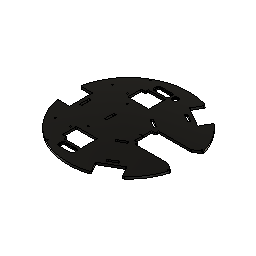
UpperPlate v16 (Autodesk Fusion 360 design; units mm, degrees)
Autodesk Fusion 360 part; units mm, degrees
(part 1 of 2)
sketch "Sketch1" plane through (0, 0, 0) normal (0, 0, 1) x (1, 0, 0)
  line L0 (0, 0) -> (-132.5, 0) construction
  line L1 (0, 0) -> (132.5, 0) construction
  line L2 (0, 0) -> (66.25, 114.7484) construction
  line L3 (0, 0) -> (66.25, -114.7484) construction
  line L4 (-130.1201, -25) -> (-103.7941, -25) construction
  line L5 (-103.7941, -25) -> (-103.7941, 25) construction
  line L6 (-103.7941, 25) -> (-130.1201, 25) construction
  line L7 (-130.1201, 25) -> (-130.1201, -25) construction
  line L8 (-103.7941, 25) -> (-104.8548, 23.9393) construction
  line L9 (-103.7941, -25) -> (-104.8548, -23.9393) construction
  arc A0 (-127.0581, -25) -> (-129.5015, -28.0288) centre (-127.0581, -27.5) ccw
  arc A1 (-129.5015, -28.0288) -> (-127.0581, -25) centre (-127.0581, -27.5) ccw construction
  arc A2 (-103.7941, -25) -> (-103.7941, -22.8787) centre (-104.8548, -23.9393) ccw
  arc A3 (-103.7941, -22.8787) -> (-105.9155, -25) centre (-104.8548, -23.9393) ccw construction
  arc A4 (-105.9155, -25) -> (-103.7941, -25) centre (-104.8548, -23.9393) ccw
  arc A5 (-103.7941, 22.8787) -> (-105.9155, 25) centre (-104.8548, 23.9393) ccw
  arc A6 (-105.9155, 25) -> (-103.7941, 22.8787) centre (-104.8548, 23.9393) ccw construction
  arc A7 (-129.5015, 28.0288) -> (-127.0581, 25) centre (-127.0581, 27.5) ccw
  arc A8 (-127.0581, 25) -> (-129.5015, 28.0288) centre (-127.0581, 27.5) ccw construction
  line L10 (-127.0581, 25) -> (-105.9155, 25)
  line L11 (-103.7941, 22.8787) -> (-103.7941, -22.8787)
  line L12 (-105.9155, -25) -> (-127.0581, -25)
  line L13 (43.4094, 125.1873) -> (86.7107, 100.1873) construction
  line L14 (43.4094, 125.1873) -> (30.2464, 102.3884) construction
  line L15 (30.2464, 102.3884) -> (73.5477, 77.3884) construction
  line L16 (73.5477, 77.3884) -> (86.7107, 100.1873) construction
  arc A9 (41.8784, 122.5355) -> (40.477, 126.166) centre (39.7133, 123.7855) ccw
  arc A10 (40.477, 126.166) -> (41.8784, 122.5355) centre (39.7133, 123.7855) ccw construction
  arc A11 (89.0244, 98.1371) -> (85.1797, 97.5355) centre (87.3447, 96.2855) ccw
  arc A12 (85.1797, 97.5355) -> (89.0244, 98.1371) centre (87.3447, 96.2855) ccw construction
  line L17 (30.2464, 102.3884) -> (31.6953, 102.7766) construction
  arc A13 (31.3071, 104.2255) -> (32.0836, 101.3277) centre (31.6953, 102.7766) ccw
  arc A14 (32.0836, 101.3277) -> (31.3071, 104.2255) centre (31.6953, 102.7766) ccw construction
  line L18 (73.5477, 77.3884) -> (73.1595, 78.8372) construction
  arc A15 (71.7106, 78.449) -> (74.6084, 79.2255) centre (73.1595, 78.8372) ccw
  arc A16 (74.6084, 79.2255) -> (71.7106, 78.449) centre (73.1595, 78.8372) ccw construction
  line L19 (74.6084, 79.2255) -> (85.1797, 97.5355)
  line L20 (71.7106, 78.449) -> (32.0836, 101.3277)
  line L21 (31.3071, 104.2255) -> (41.8784, 122.5355)
  line L22 (43.4094, -125.1873) -> (86.7107, -100.1873) construction
  line L23 (43.4094, -125.1873) -> (30.2464, -102.3884) construction
  line L24 (30.2464, -102.3884) -> (73.5477, -77.3884) construction
  line L25 (73.5477, -77.3884) -> (86.7107, -100.1873) construction
  line L26 (73.5477, -77.3884) -> (73.1595, -78.8372) construction
  line L27 (30.2464, -102.3884) -> (31.6953, -102.7766) construction
  arc A17 (32.0836, -101.3277) -> (31.3071, -104.2255) centre (31.6953, -102.7766) ccw
  arc A18 (31.3071, -104.2255) -> (32.0836, -101.3277) centre (31.6953, -102.7766) ccw construction
  arc A19 (74.6084, -79.2255) -> (71.7106, -78.449) centre (73.1595, -78.8372) ccw
  arc A20 (71.7106, -78.449) -> (74.6084, -79.2255) centre (73.1595, -78.8372) ccw construction
  arc A21 (85.1797, -97.5355) -> (89.0244, -98.1371) centre (87.3447, -96.2855) ccw
  arc A22 (89.0244, -98.1371) -> (85.1797, -97.5355) centre (87.3447, -96.2855) ccw construction
  arc A23 (40.477, -126.166) -> (41.8784, -122.5355) centre (39.7133, -123.7855) ccw
  arc A24 (41.8784, -122.5355) -> (40.477, -126.166) centre (39.7133, -123.7855) ccw construction
  line L28 (85.1797, -97.5355) -> (74.6084, -79.2255)
  line L29 (71.7106, -78.449) -> (32.0836, -101.3277)
  line L30 (31.3071, -104.2255) -> (41.8784, -122.5355)
  arc A25 (40.477, 126.166) -> (-129.5015, 28.0288) centre (0, 0) ccw
  arc A26 (-129.5015, 28.0288) -> (-129.5015, -28.0288) centre (0, 0) ccw construction
  arc A27 (40.477, -126.166) -> (40.477, 126.166) centre (0, 0) ccw construction
  arc A28 (-129.5015, -28.0288) -> (40.477, -126.166) centre (0, 0) ccw
  line L31 (-103.7941, 18.4) -> (-19.3941, 18.4) construction
  line L32 (-19.3941, 18.4) -> (-19.3941, -18.4) construction
  line L33 (-19.3941, -18.4) -> (-103.7941, -18.4) construction
  line L34 (-96.7941, 10) -> (-91.9941, 10) construction
  line L35 (-91.9941, 10) -> (-91.9941, -10) construction
  line L36 (-91.9941, -10) -> (-96.7941, -10) construction
  line L37 (-96.7941, -10) -> (-96.7941, 10) construction
  line L38 (-96.7941, 10) -> (-91.9941, -10) construction
  line L39 (-41.9941, 10) -> (-37.1941, 10) construction
  line L40 (-37.1941, 10) -> (-37.1941, -10) construction
  line L41 (-37.1941, -10) -> (-41.9941, -10) construction
  line L42 (-41.9941, -10) -> (-41.9941, 10) construction
  line L43 (-41.9941, 10) -> (-37.1941, -10) construction
  line L44 (-96.7941, 10) -> (-95.7335, 8.9393) construction
  line L45 (-91.9941, 10) -> (-93.0548, 8.9393) construction
  line L46 (-96.7941, -10) -> (-95.7335, -8.9393) construction
  line L47 (-91.9941, -10) -> (-93.0548, -8.9393) construction
  arc A29 (-94.1155, 10) -> (-91.9941, 7.8787) centre (-93.0548, 8.9393) ccw construction
  arc A30 (-91.9941, 7.8787) -> (-91.9941, 10) centre (-93.0548, 8.9393) ccw
  arc A31 (-91.9941, 10) -> (-94.1155, 10) centre (-93.0548, 8.9393) ccw
  arc A32 (-96.7941, 7.8787) -> (-94.6728, 10) centre (-95.7335, 8.9393) ccw construction
  arc A33 (-94.6728, 10) -> (-96.7941, 10) centre (-95.7335, 8.9393) ccw
  arc A34 (-96.7941, 10) -> (-96.7941, 7.8787) centre (-95.7335, 8.9393) ccw
  arc A35 (-94.6728, -10) -> (-96.7941, -7.8787) centre (-95.7335, -8.9393) ccw construction
  arc A36 (-96.7941, -7.8787) -> (-96.7941, -10) centre (-95.7335, -8.9393) ccw
  arc A37 (-96.7941, -10) -> (-94.6728, -10) centre (-95.7335, -8.9393) ccw
  arc A38 (-91.9941, -7.8787) -> (-94.1155, -10) centre (-93.0548, -8.9393) ccw construction
  arc A39 (-94.1155, -10) -> (-91.9941, -10) centre (-93.0548, -8.9393) ccw
  arc A40 (-91.9941, -10) -> (-91.9941, -7.8787) centre (-93.0548, -8.9393) ccw
  line L48 (-94.6728, 10) -> (-94.1155, 10)
  line L49 (-96.7941, 7.8787) -> (-96.7941, -7.8787)
  line L50 (-91.9941, -7.8787) -> (-91.9941, 7.8787)
  line L51 (-94.6728, -10) -> (-94.1155, -10)
  line L52 (-41.9941, 10) -> (-40.9335, 8.9393) construction
  line L53 (-37.1941, 10) -> (-38.2548, 8.9393) construction
  line L54 (-41.9941, -10) -> (-40.9335, -8.9393) construction
  line L55 (-37.1941, -10) -> (-38.2548, -8.9393) construction
  arc A41 (-37.1941, -7.8787) -> (-39.3155, -10) centre (-38.2548, -8.9393) ccw construction
  arc A42 (-39.3155, -10) -> (-37.1941, -10) centre (-38.2548, -8.9393) ccw
  arc A43 (-37.1941, -10) -> (-37.1941, -7.8787) centre (-38.2548, -8.9393) ccw
  arc A44 (-39.8728, -10) -> (-41.9941, -7.8787) centre (-40.9335, -8.9393) ccw construction
  arc A45 (-41.9941, -10) -> (-39.8728, -10) centre (-40.9335, -8.9393) ccw
  arc A46 (-41.9941, -7.8787) -> (-41.9941, -10) centre (-40.9335, -8.9393) ccw
  arc A47 (-41.9941, 7.8787) -> (-39.8728, 10) centre (-40.9335, 8.9393) ccw construction
  arc A48 (-41.9941, 10) -> (-41.9941, 7.8787) centre (-40.9335, 8.9393) ccw
  arc A49 (-39.8728, 10) -> (-41.9941, 10) centre (-40.9335, 8.9393) ccw
  arc A50 (-39.3155, 10) -> (-37.1941, 7.8787) centre (-38.2548, 8.9393) ccw construction
  arc A51 (-37.1941, 10) -> (-39.3155, 10) centre (-38.2548, 8.9393) ccw
  arc A52 (-37.1941, 7.8787) -> (-37.1941, 10) centre (-38.2548, 8.9393) ccw
  line L56 (-39.8728, -10) -> (-39.3155, -10)
  line L57 (-37.1941, -7.8787) -> (-37.1941, 7.8787)
  line L58 (-41.9941, 7.8787) -> (-41.9941, -7.8787)
  line L59 (-39.8728, 10) -> (-39.3155, 10)
  line L60 (35.9622, 99.0884) -> (-6.2378, 25.9958) construction
  line L61 (-6.2378, 25.9958) -> (25.6319, 7.5958) construction
  line L62 (25.6319, 7.5958) -> (67.8319, 80.6884) construction
  line L63 (39.7368, 88.8262) -> (57.0573, 78.8262) construction
  line L64 (57.0573, 78.8262) -> (54.6573, 74.6693) construction
  line L65 (54.6573, 74.6693) -> (37.3368, 84.6693) construction
  line L66 (37.3368, 84.6693) -> (39.7368, 88.8262) construction
  line L67 (39.7368, 88.8262) -> (54.6573, 74.6693) construction
  line L68 (12.3368, 41.368) -> (29.6573, 31.368) construction
  line L69 (29.6573, 31.368) -> (27.2573, 27.2111) construction
  line L70 (27.2573, 27.2111) -> (9.9368, 37.2111) construction
  line L71 (9.9368, 37.2111) -> (12.3368, 41.368) construction
  line L72 (12.3368, 41.368) -> (27.2573, 27.2111) construction
  line L73 (37.3368, 84.6693) -> (38.7857, 85.0575) construction
  line L74 (39.7368, 88.8262) -> (40.125, 87.3773) construction
  line L75 (54.6573, 74.6693) -> (54.2691, 76.1181) construction
  line L76 (57.0573, 78.8262) -> (55.6084, 78.438) construction
  arc A53 (55.2202, 79.8868) -> (55.9967, 76.9891) centre (55.6084, 78.438) ccw construction
  arc A54 (55.9967, 76.9891) -> (57.0573, 78.8262) centre (55.6084, 78.438) ccw
  arc A55 (57.0573, 78.8262) -> (55.2202, 79.8868) centre (55.6084, 78.438) ccw
  arc A56 (55.718, 76.5064) -> (52.8202, 75.7299) centre (54.2691, 76.1181) ccw construction
  arc A57 (54.6573, 74.6693) -> (55.718, 76.5064) centre (54.2691, 76.1181) ccw
  arc A58 (52.8202, 75.7299) -> (54.6573, 74.6693) centre (54.2691, 76.1181) ccw
  arc A59 (39.1739, 83.6086) -> (38.3975, 86.5064) centre (38.7857, 85.0575) ccw construction
  arc A60 (37.3368, 84.6693) -> (39.1739, 83.6086) centre (38.7857, 85.0575) ccw
  arc A61 (38.3975, 86.5064) -> (37.3368, 84.6693) centre (38.7857, 85.0575) ccw
  arc A62 (38.6762, 86.9891) -> (41.5739, 87.7655) centre (40.125, 87.3773) ccw construction
  arc A63 (41.5739, 87.7655) -> (39.7368, 88.8262) centre (40.125, 87.3773) ccw
  arc A64 (39.7368, 88.8262) -> (38.6762, 86.9891) centre (40.125, 87.3773) ccw
  line L77 (38.3975, 86.5064) -> (38.6762, 86.9891)
  line L78 (41.5739, 87.7655) -> (55.2202, 79.8868)
  line L79 (55.9967, 76.9891) -> (55.718, 76.5064)
  line L80 (52.8202, 75.7299) -> (39.1739, 83.6086)
  line L81 (9.9368, 37.2111) -> (11.3857, 37.5993) construction
  line L82 (12.3368, 41.368) -> (12.725, 39.9191) construction
  line L83 (27.2573, 27.2111) -> (26.8691, 28.66) construction
  line L84 (29.6573, 31.368) -> (28.2084, 30.9798) construction
  arc A65 (11.2762, 39.5309) -> (14.1739, 40.3073) centre (12.725, 39.9191) ccw construction
  arc A66 (14.1739, 40.3073) -> (12.3368, 41.368) centre (12.725, 39.9191) ccw
  arc A67 (12.3368, 41.368) -> (11.2762, 39.5309) centre (12.725, 39.9191) ccw
  arc A68 (11.7739, 36.1504) -> (10.9975, 39.0482) centre (11.3857, 37.5993) ccw construction
  arc A69 (10.9975, 39.0482) -> (9.9368, 37.2111) centre (11.3857, 37.5993) ccw
  arc A70 (9.9368, 37.2111) -> (11.7739, 36.1504) centre (11.3857, 37.5993) ccw
  arc A71 (28.318, 29.0482) -> (25.4202, 28.2717) centre (26.8691, 28.66) ccw construction
  arc A72 (25.4202, 28.2717) -> (27.2573, 27.2111) centre (26.8691, 28.66) ccw
  arc A73 (27.2573, 27.2111) -> (28.318, 29.0482) centre (26.8691, 28.66) ccw
  arc A74 (27.8202, 32.4286) -> (28.5967, 29.5309) centre (28.2084, 30.9798) ccw construction
  arc A75 (28.5967, 29.5309) -> (29.6573, 31.368) centre (28.2084, 30.9798) ccw
  arc A76 (29.6573, 31.368) -> (27.8202, 32.4286) centre (28.2084, 30.9798) ccw
  line L85 (10.9975, 39.0482) -> (11.2762, 39.5309)
  line L86 (11.7739, 36.1504) -> (25.4202, 28.2717)
  line L87 (28.318, 29.0482) -> (28.5967, 29.5309)
  line L88 (27.8202, 32.4286) -> (14.1739, 40.3073)
  line L89 (35.9622, -99.0884) -> (-6.2378, -25.9958) construction
  line L90 (-6.2378, -25.9958) -> (25.6319, -7.5958) construction
  line L91 (25.6319, -7.5958) -> (67.8319, -80.6884) construction
  line L92 (39.7368, -88.8262) -> (57.0573, -78.8262) construction
  line L93 (57.0573, -78.8262) -> (54.6573, -74.6693) construction
  line L94 (54.6573, -74.6693) -> (37.3368, -84.6693) construction
  line L95 (37.3368, -84.6693) -> (39.7368, -88.8262) construction
  line L96 (37.3368, -84.6693) -> (57.0573, -78.8262) construction
  line L97 (12.3368, -41.368) -> (29.6573, -31.368) construction
  line L98 (29.6573, -31.368) -> (27.2573, -27.2111) construction
  line L99 (27.2573, -27.2111) -> (9.9368, -37.2111) construction
  line L100 (9.9368, -37.2111) -> (12.3368, -41.368) construction
  line L101 (9.9368, -37.2111) -> (29.6573, -31.368) construction
  line L102 (9.9368, -37.2111) -> (11.3857, -37.5993) construction
  line L103 (12.3368, -41.368) -> (12.725, -39.9191) construction
  line L104 (27.2573, -27.2111) -> (26.8691, -28.66) construction
  line L105 (29.6573, -31.368) -> (28.2084, -30.9798) construction
  arc A77 (25.4202, -28.2717) -> (28.318, -29.0482) centre (26.8691, -28.66) ccw construction
  arc A78 (28.318, -29.0482) -> (27.2573, -27.2111) centre (26.8691, -28.66) ccw
  arc A79 (27.2573, -27.2111) -> (25.4202, -28.2717) centre (26.8691, -28.66) ccw
  arc A80 (28.5967, -29.5309) -> (27.8202, -32.4286) centre (28.2084, -30.9798) ccw construction
  arc A81 (29.6573, -31.368) -> (28.5967, -29.5309) centre (28.2084, -30.9798) ccw
  arc A82 (27.8202, -32.4286) -> (29.6573, -31.368) centre (28.2084, -30.9798) ccw
  arc A83 (14.1739, -40.3073) -> (11.2762, -39.5309) centre (12.725, -39.9191) ccw construction
  arc A84 (12.3368, -41.368) -> (14.1739, -40.3073) centre (12.725, -39.9191) ccw
  arc A85 (11.2762, -39.5309) -> (12.3368, -41.368) centre (12.725, -39.9191) ccw
  arc A86 (10.9975, -39.0482) -> (11.7739, -36.1504) centre (11.3857, -37.5993) ccw construction
  arc A87 (9.9368, -37.2111) -> (10.9975, -39.0482) centre (11.3857, -37.5993) ccw
  arc A88 (11.7739, -36.1504) -> (9.9368, -37.2111) centre (11.3857, -37.5993) ccw
  line L106 (28.5967, -29.5309) -> (28.318, -29.0482)
  line L107 (25.4202, -28.2717) -> (11.7739, -36.1504)
  line L108 (27.8202, -32.4286) -> (14.1739, -40.3073)
  line L109 (11.2762, -39.5309) -> (10.9975, -39.0482)
  line L110 (37.3368, -84.6693) -> (38.7857, -85.0575) construction
  line L111 (39.7368, -88.8262) -> (40.125, -87.3773) construction
  line L112 (54.6573, -74.6693) -> (54.2691, -76.1181) construction
  line L113 (57.0573, -78.8262) -> (55.6084, -78.438) construction
  arc A89 (38.3975, -86.5064) -> (39.1739, -83.6086) centre (38.7857, -85.0575) ccw construction
  arc A90 (39.1739, -83.6086) -> (37.3368, -84.6693) centre (38.7857, -85.0575) ccw
  arc A91 (37.3368, -84.6693) -> (38.3975, -86.5064) centre (38.7857, -85.0575) ccw
  arc A92 (41.5739, -87.7655) -> (38.6762, -86.9891) centre (40.125, -87.3773) ccw construction
  arc A93 (38.6762, -86.9891) -> (39.7368, -88.8262) centre (40.125, -87.3773) ccw
  arc A94 (39.7368, -88.8262) -> (41.5739, -87.7655) centre (40.125, -87.3773) ccw
  arc A95 (55.9967, -76.9891) -> (55.2202, -79.8868) centre (55.6084, -78.438) ccw construction
  arc A96 (55.2202, -79.8868) -> (57.0573, -78.8262) centre (55.6084, -78.438) ccw
  arc A97 (57.0573, -78.8262) -> (55.9967, -76.9891) centre (55.6084, -78.438) ccw
  arc A98 (52.8202, -75.7299) -> (55.718, -76.5064) centre (54.2691, -76.1181) ccw construction
  arc A99 (55.718, -76.5064) -> (54.6573, -74.6693) centre (54.2691, -76.1181) ccw
  arc A100 (54.6573, -74.6693) -> (52.8202, -75.7299) centre (54.2691, -76.1181) ccw
  line L114 (38.6762, -86.9891) -> (38.3975, -86.5064)
  line L115 (39.1739, -83.6086) -> (52.8202, -75.7299)
  line L116 (55.718, -76.5064) -> (55.9967, -76.9891)
  line L117 (55.2202, -79.8868) -> (41.5739, -87.7655)
  line L118 (32, 18.3) -> (131.2302, 18.3) construction
  line L119 (131.2302, 18.3) -> (131.2302, -18.3) construction
  line L120 (131.2302, -18.3) -> (32, -18.3) construction
  line L121 (32, -18.3) -> (32, 18.3) construction
  line L122 (40, 25.5) -> (130.0231, 25.5) construction
  line L123 (130.0231, 25.5) -> (130.0231, -25.5) construction
  line L124 (130.0231, -25.5) -> (40, -25.5) construction
  line L125 (40, -25.5) -> (40, 25.5) construction
  line L126 (105, 25.5) -> (105, -25.5) construction
  line L127 (105, 22.5) -> (127.6365, 35.5692) construction
  line L128 (105, -22.5) -> (127.6365, -35.5692) construction
  line L129 (32, -18.3) -> (33.0607, -17.2393) construction
  line L130 (40, -25.5) -> (41.0607, -24.4393) construction
  circle A101 centre (33.0607, -17.2393) radius 1.5 construction
  circle A102 centre (41.0607, -24.4393) radius 1.5 construction
  circle A103 centre (37.5, -20.8) radius 2.5 construction
  line L131 (32, 18.3) -> (33.0607, 17.2393) construction
  line L132 (40, 25.5) -> (41.0607, 24.4393) construction
  circle A104 centre (41.0607, 24.4393) radius 1.5 construction
  circle A105 centre (33.0607, 17.2393) radius 1.5 construction
  circle A106 centre (37.5, 20.8) radius 2.5 construction
  circle A107 centre (124.6951, -36.7577) radius 2.5 construction
  circle A108 centre (124.6951, 36.7577) radius 2.5 construction
  circle A109 centre (109.5263, 28) radius 2.5 construction
  circle A110 centre (109.5263, -28) radius 2.5 construction
  line L133 (32, 16.1787) -> (32, -16.1787)
  line L134 (34.1213, -18.3) -> (37.5, -18.3)
  line L135 (40, -20.8) -> (40, -23.3787)
  line L136 (42.1213, -25.5) -> (109.5263, -25.5)
  line L137 (110.7763, -25.8349) -> (125.9451, -34.5927)
  line L138 (34.1213, 18.3) -> (37.5, 18.3)
  line L139 (40, 20.8) -> (40, 23.3787)
  line L140 (42.1213, 25.5) -> (109.5263, 25.5)
  line L141 (110.7763, 25.8349) -> (125.9451, 34.5927)
  arc A111 (34.1213, 18.3) -> (32, 16.1787) centre (33.0607, 17.2393) ccw
  arc A112 (42.1213, 25.5) -> (40, 23.3787) centre (41.0607, 24.4393) ccw
  arc A113 (32, -16.1787) -> (34.1213, -18.3) centre (33.0607, -17.2393) ccw
  arc A114 (40, -23.3787) -> (42.1213, -25.5) centre (41.0607, -24.4393) ccw
  arc A115 (37.5, 18.3) -> (40, 20.8) centre (37.5, 20.8) ccw
  arc A116 (40, -20.8) -> (37.5, -18.3) centre (37.5, -20.8) ccw
  arc A117 (109.5263, 25.5) -> (110.7763, 25.8349) centre (109.5263, 28) ccw
  arc A118 (110.7763, -25.8349) -> (109.5263, -25.5) centre (109.5263, -28) ccw
  line L142 (0, 0) -> (124.6951, -36.7577) construction
  line L143 (124.6951, -36.7577) -> (127.0931, -37.4646) construction
  arc A119 (127.0931, -37.4646) -> (125.9451, -34.5927) centre (124.6951, -36.7577) ccw
  line L144 (0, 0) -> (124.6951, 36.7577) construction
  line L145 (124.6951, 36.7577) -> (127.0931, 37.4646) construction
  arc A120 (125.9451, 34.5927) -> (127.0931, 37.4646) centre (124.6951, 36.7577) ccw
  arc A121 (89.0244, -98.1371) -> (127.0931, -37.4646) centre (0, 0) ccw
  arc A122 (127.0931, 37.4646) -> (89.0244, 98.1371) centre (0, 0) ccw
  line L146 (127.6365, -35.5692) -> (123.5112, -37.2289) construction
  circle A123 centre (123.5112, -37.2289) radius 3.5 construction
  circle A124 centre (123.5112, -37.2289) radius 1.5
  line L147 (86.7107, -100.1873) -> (87.5879, -94.7067) construction
  circle A125 centre (87.5879, -94.7067) radius 3.5 construction
  circle A126 centre (87.5879, -94.7067) radius 1.5 construction
  line L148 (43.4094, -125.1873) -> (38.2245, -123.2067) construction
  circle A127 centre (38.2245, -123.2067) radius 3.5 construction
  circle A128 centre (38.2245, -123.2067) radius 1.5 construction
  line L149 (-130.1201, -25) -> (-125.8124, -28.5) construction
  circle A129 centre (-125.8124, -28.5) radius 3.5 construction
  circle A130 centre (-125.8124, -28.5) radius 1.5 construction
  line L150 (-130.1201, 25) -> (-125.8124, 28.5) construction
  circle A131 centre (-125.8124, 28.5) radius 3.5 construction
  circle A132 centre (-125.8124, 28.5) radius 1.5 construction
  line L151 (43.4094, 125.1873) -> (38.2245, 123.2067) construction
  circle A133 centre (38.2245, 123.2067) radius 3.5 construction
  circle A134 centre (38.2245, 123.2067) radius 1.5 construction
  line L152 (86.7107, 100.1873) -> (87.5879, 94.7067) construction
  circle A135 centre (87.5879, 94.7067) radius 3.5 construction
  circle A136 centre (87.5879, 94.7067) radius 1.5 construction
  line L153 (127.6365, 35.5692) -> (123.5112, 37.2289) construction
  circle A137 centre (123.5112, 37.2289) radius 3.5 construction
  circle A138 centre (123.5112, 37.2289) radius 1.5
  line L154 (-125.8124, -28.5) -> (38.2245, -123.2067) construction
  line L155 (-125.8124, 28.5) -> (38.2245, 123.2067) construction
  line L156 (0, 0) -> (-43.794, -75.8534) construction
  line L157 (-43.794, -75.8534) -> (-64.5, -111.7173) construction
  circle A139 centre (-64.5, -111.7173) radius 3.5 construction
  circle A140 centre (-64.5, -111.7173) radius 1.5
  line L158 (0, 0) -> (-43.794, 75.8534) construction
  line L159 (-43.794, 75.8534) -> (-64.5, 111.7173) construction
  circle A141 centre (-64.5, 111.7173) radius 3.5 construction
  circle A142 centre (-64.5, 111.7173) radius 1.5
  line L160 (32.0836, -101.3277) -> (21.5862, -107.3884) construction
  line L161 (21.5862, -107.3884) -> (33.586, -128.1727) construction
  circle A143 centre (28.2185, -125.8758) radius 3.5 construction
  circle A144 centre (28.2185, -125.8758) radius 1.5
  line L162 (71.7106, -78.449) -> (82.208, -72.3884) construction
  line L163 (82.208, -72.3884) -> (94.2078, -93.1727) construction
  circle A145 centre (94.9024, -87.3758) radius 3.5 construction
  line L164 (-103.7941, -25) -> (-103.7941, -35) construction
  line L165 (-103.7941, -35) -> (-127.7938, -35) construction
  circle A146 centre (-123.1209, -38.5) radius 3.5 construction
  line L166 (-103.7941, 25) -> (-103.7941, 35) construction
  line L167 (-103.7941, 35) -> (-127.7938, 35) construction
  circle A147 centre (-123.1209, 38.5) radius 3.5 construction
  line L168 (30.2464, 102.3884) -> (21.5862, 107.3884) construction
  line L169 (21.5862, 107.3884) -> (33.586, 128.1727) construction
  circle A148 centre (28.2185, 125.8758) radius 3.5 construction
  line L170 (73.5477, 77.3884) -> (82.208, 72.3884) construction
  line L171 (82.208, 72.3884) -> (94.2078, 93.1727) construction
  circle A149 centre (94.9024, 87.3758) radius 3.5 construction
  circle A150 centre (94.9024, 87.3758) radius 1.5
  circle A151 centre (28.2185, 125.8758) radius 1.5
  circle A152 centre (-123.1209, 38.5) radius 1.5
  circle A153 centre (-123.1209, -38.5) radius 1.5
  circle A154 centre (94.9024, -87.3758) radius 1.5
  line L172 (-103.7941, 56) -> (12.8059, 56) construction
  line L173 (12.8059, 56) -> (12.8059, -56) construction
  line L174 (12.8059, -56) -> (-103.7941, -56) construction
  line L175 (-103.7941, -56) -> (-103.7941, 56) construction
  circle A155 centre (-86.2941, -31.5) radius 4.25 construction
  circle A156 centre (-45.4941, 42.5) radius 1.5
  line L176 (-45.4941, 42.5) -> (-45.4941, -42.5) construction
  circle A157 centre (-45.4941, -42.5) radius 1.5
  line L177 (-10.1941, 76) -> (-3.6941, 76) construction
  line L178 (-3.6941, 76) -> (-3.6941, 56) construction
  line L179 (-3.6941, 56) -> (-10.1941, 56) construction
  line L180 (-10.1941, 56) -> (-10.1941, 76) construction
  line L181 (-48.7941, 92) -> (-11.7941, 92) construction
  line L182 (-11.7941, 92) -> (-11.7941, 56) construction
  line L183 (-11.7941, 56) -> (-48.7941, 56) construction
  line L184 (-48.7941, 56) -> (-48.7941, 92) construction
  line L185 (-48.7941, -56) -> (-11.7941, -56) construction
  line L186 (-11.7941, -56) -> (-11.7941, -92) construction
  line L187 (-11.7941, -92) -> (-48.7941, -92) construction
  line L188 (-48.7941, -92) -> (-48.7941, -56) construction
  line L189 (-57.7941, -56) -> (-57.7941, -86) construction
  line L190 (-57.7941, -86) -> (-48.7941, -86) construction
  line L191 (-48.7941, 86) -> (-57.7941, 86) construction
  line L192 (-57.7941, 86) -> (-57.7941, 56) construction
  circle A158 centre (-50.2941, 87.5) radius 1.5 construction
  line L193 (-50.2941, 87.5) -> (-50.2941, 86) construction
  line L194 (-50.2941, 87.5) -> (-48.7941, 87.5) construction
  circle A159 centre (-50.2941, -87.5) radius 1.5 construction
  line L195 (-50.2941, -87.5) -> (-50.2941, -86) construction
  line L196 (-50.2941, -87.5) -> (-48.7941, -87.5) construction
  line L197 (-57.7941, -86) -> (-56.7335, -84.9393) construction
  line L198 (-48.7941, -92) -> (-47.7335, -90.9393) construction
  circle A160 centre (-56.7335, -84.9393) radius 1.5 construction
  circle A161 centre (-47.7335, -90.9393) radius 1.5 construction
  line L199 (-57.7941, -56) -> (-56.7335, -57.0607) construction
  circle A162 centre (-56.7335, -57.0607) radius 1.5 construction
  line L200 (-11.7941, -56) -> (-12.8548, -57.0607) construction
  circle A163 centre (-12.8548, -57.0607) radius 1.5 construction
  line L201 (-11.7941, -92) -> (-12.8548, -90.9393) construction
  circle A164 centre (-12.8548, -90.9393) radius 1.5 construction
  line L202 (-57.7941, 86) -> (-56.7335, 84.9393) construction
  line L203 (-48.7941, 92) -> (-47.7335, 90.9393) construction
  line L204 (-11.7941, 92) -> (-12.8548, 90.9393) construction
  circle A165 centre (-56.7335, 84.9393) radius 1.5 construction
  circle A166 centre (-47.7335, 90.9393) radius 1.5 construction
  circle A167 centre (-12.8548, 90.9393) radius 1.5 construction
  line L205 (-57.7941, 56) -> (-56.7335, 57.0607) construction
  line L206 (-11.7941, 56) -> (-12.8548, 57.0607) construction
  circle A168 centre (-12.8548, 57.0607) radius 1.5 construction
  circle A169 centre (-56.7335, 57.0607) radius 1.5 construction
  line L207 (-57.7941, 58.1213) -> (-57.7941, 83.8787)
  line L208 (-55.6728, 56) -> (-13.9155, 56)
  line L209 (-11.7941, 58.1213) -> (-11.7941, 89.8787)
  line L210 (-13.9155, 92) -> (-46.6728, 92)
  line L211 (-48.7941, 89.8787) -> (-48.7941, 87.5)
  line L212 (-50.2941, 86) -> (-55.6728, 86)
  arc A170 (-46.6728, 92) -> (-48.7941, 89.8787) centre (-47.7335, 90.9393) ccw
  arc A171 (-50.2941, 86) -> (-48.7941, 87.5) centre (-50.2941, 87.5) ccw
  arc A172 (-55.6728, 86) -> (-57.7941, 83.8787) centre (-56.7335, 84.9393) ccw
  arc A173 (-11.7941, 89.8787) -> (-13.9155, 92) centre (-12.8548, 90.9393) ccw
  arc A174 (-13.9155, 56) -> (-11.7941, 58.1213) centre (-12.8548, 57.0607) ccw
  arc A175 (-57.7941, 58.1213) -> (-55.6728, 56) centre (-56.7335, 57.0607) ccw
  line L213 (-57.7941, -58.1213) -> (-57.7941, -83.8787)
  line L214 (-55.6728, -86) -> (-50.2941, -86)
  line L215 (-48.7941, -87.5) -> (-48.7941, -89.8787)
  line L216 (-46.6728, -92) -> (-13.9155, -92)
  line L217 (-11.7941, -89.8787) -> (-11.7941, -58.1213)
  line L218 (-13.9155, -56) -> (-55.6728, -56)
  arc A176 (-55.6728, -56) -> (-57.7941, -58.1213) centre (-56.7335, -57.0607) ccw
  arc A177 (-11.7941, -58.1213) -> (-13.9155, -56) centre (-12.8548, -57.0607) ccw
  arc A178 (-57.7941, -83.8787) -> (-55.6728, -86) centre (-56.7335, -84.9393) ccw
  arc A179 (-48.7941, -87.5) -> (-50.2941, -86) centre (-50.2941, -87.5) ccw
  arc A180 (-48.7941, -89.8787) -> (-46.6728, -92) centre (-47.7335, -90.9393) ccw
  arc A181 (-13.9155, -92) -> (-11.7941, -89.8787) centre (-12.8548, -90.9393) ccw
  line L219 (-41.8941, -97) -> (-15.4941, -97)
  line L220 (-11.7941, -100.7) -> (-11.7941, -107.7)
  line L221 (-15.4941, -111.4) -> (-41.8941, -111.4)
  line L222 (-45.5941, -107.7) -> (-45.5941, -100.7)
  line L223 (-11.7941, -92) -> (-11.7941, -97)
  arc A182 (-41.8941, -97) -> (-45.5941, -100.7) centre (-41.8941, -100.7) ccw
  arc A183 (-11.7941, -100.7) -> (-15.4941, -97) centre (-15.4941, -100.7) ccw
  arc A184 (-45.5941, -107.7) -> (-41.8941, -111.4) centre (-41.8941, -107.7) ccw
  arc A185 (-15.4941, -111.4) -> (-11.7941, -107.7) centre (-15.4941, -107.7) ccw
  line L224 (-43.7441, -98.65) -> (-13.6441, -98.65) construction
  line L225 (-13.6441, -98.65) -> (-13.6441, -109.75) construction
  line L226 (-13.6441, -109.75) -> (-43.7441, -109.75) construction
  line L227 (-43.7441, -109.75) -> (-43.7441, -98.65) construction
  line L228 (-43.7441, -98.65) -> (-42.6835, -99.7107) construction
  line L229 (-13.6441, -98.65) -> (-14.7048, -99.7107) construction
  line L230 (-43.7441, -109.75) -> (-42.6835, -108.6893) construction
  line L231 (-13.6441, -109.75) -> (-14.7048, -108.6893) construction
  circle A186 centre (-42.6835, -99.7107) radius 1.5 construction
  circle A187 centre (-42.6835, -108.6893) radius 1.5 construction
  circle A188 centre (-14.7048, -99.7107) radius 1.5 construction
  circle A189 centre (-14.7048, -108.6893) radius 1.5 construction
  line L232 (-41.6228, -98.65) -> (-15.7655, -98.65)
  line L233 (-43.7441, -100.7713) -> (-43.7441, -107.6287)
  line L234 (-41.6228, -109.75) -> (-15.7655, -109.75)
  line L235 (-13.6441, -107.6287) -> (-13.6441, -100.7713)
  arc A190 (-13.6441, -100.7713) -> (-15.7655, -98.65) centre (-14.7048, -99.7107) ccw
  arc A191 (-15.7655, -109.75) -> (-13.6441, -107.6287) centre (-14.7048, -108.6893) ccw
  arc A192 (-43.7441, -107.6287) -> (-41.6228, -109.75) centre (-42.6835, -108.6893) ccw
  arc A193 (-41.6228, -98.65) -> (-43.7441, -100.7713) centre (-42.6835, -99.7107) ccw
  line L236 (-41.8941, 111.4) -> (-15.4941, 111.4) construction
  line L237 (-11.7941, 107.7) -> (-11.7941, 97) construction
  line L238 (-11.7941, 97) -> (-41.8941, 97) construction
  line L239 (-45.5941, 100.7) -> (-45.5941, 107.7) construction
  line L240 (-11.7941, 92) -> (-11.7941, 97) construction
  arc A194 (-41.8941, 111.4) -> (-45.5941, 107.7) centre (-41.8941, 107.7) ccw construction
  arc A195 (-11.7941, 107.7) -> (-15.4941, 111.4) centre (-15.4941, 107.7) ccw construction
  arc A196 (-45.5941, 100.7) -> (-41.8941, 97) centre (-41.8941, 100.7) ccw construction
  circle A197 centre (-1.7941, 104.2) radius 5.5
  line L241 (-45.5941, 104.2) -> (-11.7941, 104.2) construction
  line L242 (-11.7941, 104.2) -> (-1.7941, 104.2) construction
  point P0 (-19.3941, 0)
  point P1 (-94.3941, 0)
  point P2 (-39.5941, 0)
  point P3 (9.6971, 16.7958)
  point P4 (47.1971, 81.7477)
  point P5 (19.7971, 34.2895)
  point P6 (9.6971, -16.7958)
  point P7 (47.1971, -81.7477)
  point P8 (19.7971, -34.2895)
  point P9 (-43.794, 75.8534)
  point P10 (-43.794, -75.8534)
  point P11 (12.8059, 0)
  point P12 (-45.5941, -97)
  point P13 (-11.7941, -97)
  point P14 (-45.5941, -111.4)
  point P15 (-45.5941, 111.4)
  point P16 (-11.7941, 111.4)
  point P17 (-45.5941, 97)
  dimension "d1" = 265
  dimension "d2" = 60
  dimension "d3" = 60
  dimension "d4" = 26.326
  dimension "d5" = 50
  dimension "d6" = 5
  dimension "d7" = 1.5
  dimension "d8" = 45
  dimension "d9" = 1.5
  dimension "d10" = 45
  dimension "d11" = 5
  dimension "d12" = 50
  dimension "d13" = 26.326
  dimension "d14" = 5
  dimension "d15" = 5
  dimension "d16" = 1.5
  dimension "d17" = 45
  dimension "d18" = 1.5
  dimension "d19" = 45
  dimension "d21" = 50
  dimension "d22" = 26.326
  dimension "d23" = 5
  dimension "d24" = 5
  dimension "d25" = 1.5
  dimension "d26" = 45
  dimension "d27" = 1.5
  dimension "d28" = 45
  dimension "d29" = 36.8
  dimension "d30" = 110.726
  dimension "d31" = 4.8
  dimension "d32" = 20
  dimension "d34" = 72.6
  dimension "d35" = 4.8
  dimension "d36" = 20
  dimension "d37" = 50
  dimension "d38" = 1.5
  dimension "d39" = 1.5
  dimension "d40" = 1.5
  dimension "d41" = 1.5
  dimension "d42" = 45
  dimension "d43" = 45
  dimension "d44" = 45
  dimension "d45" = 45
  dimension "d46" = 1.5
  dimension "d47" = 1.5
  dimension "d48" = 1.5
  dimension "d49" = 1.5
  dimension "d50" = 45
  dimension "d51" = 45
  dimension "d52" = 45
  dimension "d53" = 45
  dimension "d54" = 36.8
  dimension "d55" = 110.726
  dimension "d56" = 4.8
  dimension "d57" = 20
  dimension "d58" = 72.6
  dimension "d59" = 4.8
  dimension "d60" = 20
  dimension "d61" = 50
  dimension "d62" = 1.5
  dimension "d63" = 1.5
  dimension "d64" = 1.5
  dimension "d65" = 1.5
  dimension "d66" = 45
  dimension "d67" = 45
  dimension "d68" = 45
  dimension "d69" = 45
  dimension "d70" = 1.5
  dimension "d71" = 1.5
  dimension "d72" = 1.5
  dimension "d73" = 1.5
  dimension "d74" = 45
  dimension "d75" = 45
  dimension "d76" = 45
  dimension "d77" = 45
  dimension "d78" = 36.8
  dimension "d79" = 110.726
  dimension "d81" = 4.8
  dimension "d82" = 20
  dimension "d83" = 72.6
  dimension "d84" = 4.8
  dimension "d85" = 20
  dimension "d86" = 50
  dimension "d87" = 1.5
  dimension "d88" = 1.5
  dimension "d89" = 1.5
  dimension "d90" = 1.5
  dimension "d91" = 45
  dimension "d92" = 45
  dimension "d93" = 45
  dimension "d94" = 45
  dimension "d95" = 1.5
  dimension "d96" = 1.5
  dimension "d97" = 1.5
  dimension "d98" = 1.5
  dimension "d99" = 45
  dimension "d100" = 45
  dimension "d101" = 45
  dimension "d102" = 45
  dimension "d103" = 36.6
  dimension "d104" = 32
  dimension "d105" = 8
  dimension "d106" = 51
  dimension "d107" = 65
  dimension "d108" = 3
  dimension "d109" = 30
  dimension "d110" = 3
  dimension "d111" = 30
  dimension "d112" = 1.5
  dimension "d113" = 1.5
  dimension "d114" = 45
  dimension "d115" = 45
  dimension "d116" = 5
  dimension "d117" = 1.5
  dimension "d118" = 1.5
  dimension "d119" = 45
  dimension "d120" = 45
  dimension "d121" = 5
  dimension "d122" = 5
  dimension "d123" = 5
  dimension "d124" = 5
  dimension "d125" = 5
  dimension "d131" = 7
  dimension "d132" = 3
  dimension "d133" = 7
  dimension "d134" = 3
  dimension "d135" = 7
  dimension "d136" = 3
  dimension "d137" = 7
  dimension "d138" = 3
  dimension "d139" = 7
  dimension "d140" = 3
  dimension "d141" = 7
  dimension "d142" = 3
  dimension "d143" = 7
  dimension "d144" = 3
  dimension "d145" = 7
  dimension "d146" = 3
  dimension "d147" = 7
  dimension "d148" = 3
  dimension "d149" = 7
  dimension "d150" = 3
  dimension "d151" = 10
  dimension "d152" = 7
  dimension "d153" = 3
  dimension "d154" = 10
  dimension "d155" = 7
  dimension "d156" = 10
  dimension "d157" = 7
  dimension "d158" = 10
  dimension "d159" = 7
  dimension "d160" = 10
  dimension "d161" = 7
  dimension "d162" = 10
  dimension "d163" = 7
  dimension "d164" = 3
  dimension "d165" = 3
  dimension "d166" = 3
  dimension "d167" = 3
  dimension "d168" = 3
  dimension "d169" = 116.6
  dimension "d170" = 112
  dimension "d171" = 8.5
  dimension "d172" = 17.5
  dimension "d173" = 24.5
  dimension "d174" = 3
  dimension "d175" = 3
  dimension "d176" = 85
  dimension "d177" = 58.3
  dimension "d178" = 13.5
  dimension "d179" = 20
  dimension "d180" = 6.5
  dimension "d181" = 16.5
  dimension "d182" = 36
  dimension "d183" = 37
  dimension "d184" = 55
  dimension "d185" = 37
  dimension "d186" = 36
  dimension "d187" = 55
  dimension "d188" = 46
  dimension "d189" = 30
  dimension "d190" = 30
  dimension "d191" = 46
  dimension "d192" = 3
  dimension "d193" = 3
  dimension "d194" = 1.5
  dimension "d195" = 1.5
  dimension "d196" = 45
  dimension "d197" = 45
  dimension "d198" = 1.5
  dimension "d199" = 45
  dimension "d200" = 1.5
  dimension "d201" = 45
  dimension "d202" = 1.5
  dimension "d203" = 45
  dimension "d204" = 1.5
  dimension "d205" = 1.5
  dimension "d206" = 1.5
  dimension "d207" = 45
  dimension "d208" = 45
  dimension "d209" = 45
  dimension "d210" = 1.5
  dimension "d211" = 1.5
  dimension "d212" = 45
  dimension "d213" = 45
  dimension "d214" = 33.8
  dimension "d215" = 14.4
  dimension "d216" = 5
  dimension "d217" = 3.7
  dimension "d218" = 3.7
  dimension "d219" = 3.7
  dimension "d220" = 3.7
  dimension "d221" = 30.1
  dimension "d222" = 11.1
  dimension "d223" = 1.85
  dimension "d224" = 1.65
  dimension "d225" = 1.5
  dimension "d226" = 1.5
  dimension "d227" = 1.5
  dimension "d228" = 1.5
  dimension "d229" = 45
  dimension "d230" = 45
  dimension "d231" = 45
  dimension "d232" = 45
  dimension "d233" = 33.8
  dimension "d234" = 14.4
  dimension "d235" = 5
  dimension "d236" = 3.7
  dimension "d237" = 3.7
  dimension "d238" = 3.7
  dimension "d272" = 11
  dimension "d303" = 10
  constraint coincident L0.start L1.start
  constraint coincident L0.end A26
  constraint horizontal L0
  constraint coincident L1.end A26
  constraint parallel L0 L1
  constraint coincident L2.end A26
  constraint coincident L3.end A26
  constraint horizontal L4
  constraint vertical L5
  constraint horizontal L6
  constraint vertical L7
  constraint coincident L4.start A26
  constraint coincident L6.end A26
  constraint tangent L6 A7
  constraint tangent A7 A26
  constraint coincident L8.end A5.centre
  constraint coincident L5.end A5
  constraint coincident L9.end A2.centre
  constraint tangent L4 A0
  constraint tangent A0 A26
  constraint coincident L4 A0.start
  constraint concentric A0 A1
  constraint coincident L5 A2.end
  constraint coincident L4 A3.end
  constraint concentric A2 A3
  constraint concentric A2 A4
  constraint coincident L6 A5.end
  constraint coincident L5 A5.start
  constraint concentric A5 A6
  constraint coincident L6 A7.end
  constraint concentric A7 A8
  constraint coincident L13.start A26
  constraint coincident L13.end A26
  constraint perpendicular L2 L13
  constraint perpendicular L13 L14
  constraint perpendicular L14 L15
  constraint perpendicular L15 L16
  constraint tangent L14 A9
  constraint tangent A9 A26
  constraint coincident L14 A9.start
  constraint concentric A9 A10
  constraint tangent A11 A26
  constraint tangent L16 A11
  constraint coincident L16 A11.end
  constraint coincident A11.start A26
  constraint concentric A11 A12
  constraint coincident L17.end A13.centre
  constraint coincident L14.end A13
  constraint coincident L15 A13.end
  constraint coincident L14 A13.start
  constraint concentric A13 A14
  constraint coincident L18.end A15.centre
  constraint coincident L15.end A15
  constraint coincident L16 A15.end
  constraint coincident L15 A15.start
  constraint concentric A15 A16
  constraint coincident L22.start A26
  constraint coincident L22.end A26
  constraint perpendicular L3 L22
  constraint perpendicular L22 L23
  constraint perpendicular L23 L24
  constraint perpendicular L24 L25
  constraint tangent L23 A23
  constraint tangent A23 A26
  constraint tangent L25 A21
  constraint tangent A21 A26
  constraint coincident L26.end A19.centre
  constraint coincident L24.end A19
  constraint coincident L27.end A17.centre
  constraint coincident L23.end A17
  constraint coincident L23 A17.end
  constraint coincident L24 A17.start
  constraint concentric A17 A18
  constraint coincident L24 A19.end
  constraint coincident L25 A19.start
  constraint concentric A19 A20
  constraint coincident A21.end A26
  constraint coincident L25 A21.start
  constraint concentric A21 A22
  constraint coincident L23 A23.end
  constraint coincident A23.start A26
  constraint concentric A23 A24
  constraint coincident A21 A22.end
  constraint concentric A25 A26
  constraint concentric A26 A27
  constraint concentric A26 A28
  constraint coincident L11 L31.start
  constraint perpendicular L11 L31
  constraint perpendicular L31 L32
  constraint coincident L11 L33.end
  constraint perpendicular L32 L33
  constraint midpoint L32 P0
  constraint coincident L0 P0
  constraint horizontal L34
  constraint vertical L35
  constraint horizontal L36
  constraint vertical L37
  constraint midpoint L38 P1
  constraint coincident L0 P1
  constraint horizontal L39
  constraint vertical L40
  constraint horizontal L41
  constraint vertical L42
  constraint midpoint L43 P2
  constraint coincident L0 P2
  constraint coincident L44.end A32.centre
  constraint coincident L45.end A29.centre
  constraint coincident L46.end A35.centre
  constraint coincident L47.end A38.centre
  constraint coincident L35 A29.end
  constraint concentric A29 A30
  constraint coincident L34 A29.start
  constraint concentric A29 A31
  constraint coincident L34 A32.end
  constraint concentric A32 A33
  constraint coincident L37 A32.start
  constraint concentric A32 A34
  constraint coincident L37 A35.end
  constraint concentric A35 A36
  constraint coincident L36 A35.start
  constraint concentric A35 A37
  constraint coincident L36 A38.end
  constraint concentric A38 A39
  constraint coincident L35 A38.start
  constraint concentric A38 A40
  constraint coincident L54.end A44.centre
  constraint coincident L55.end A41.centre
  constraint coincident L52.end A47.centre
  constraint coincident L53.end A50.centre
  constraint coincident L41 A41.end
  constraint concentric A41 A42
  constraint coincident L40 A41.start
  constraint concentric A41 A43
  constraint coincident L41 A44.start
  constraint concentric A44 A45
  constraint coincident L42 A44.end
  constraint concentric A44 A46
  constraint coincident L42 A47.start
  constraint concentric A47 A48
  constraint coincident L39 A47.end
  constraint concentric A47 A49
  constraint coincident L39 A50.start
  constraint concentric A50 A51
  constraint coincident L40 A50.end
  constraint concentric A50 A52
  constraint coincident L20 L60.start
  constraint perpendicular L20 L60
  constraint perpendicular L60 L61
  constraint coincident L20 L62.end
  constraint perpendicular L61 L62
  constraint midpoint L61 P3
  constraint coincident L2 P3
  constraint perpendicular L2 L63
  constraint perpendicular L63 L64
  constraint perpendicular L64 L65
  constraint perpendicular L65 L66
  constraint midpoint L67 P4
  constraint coincident L2 P4
  constraint perpendicular L2 L68
  constraint perpendicular L68 L69
  constraint perpendicular L2 L70
  constraint perpendicular L70 L71
  constraint midpoint L72 P5
  constraint coincident L2 P5
  constraint coincident L74.end A62.centre
  constraint coincident L73.end A59.centre
  constraint coincident L76.end A53.centre
  constraint coincident L75.end A56.centre
  constraint coincident L64 A53.end
  constraint concentric A53 A54
  constraint coincident L63 A53.start
  constraint concentric A53 A55
  constraint coincident L64 A56.start
  constraint concentric A56 A57
  constraint coincident L65 A56.end
  constraint concentric A56 A58
  constraint coincident L65 A59.start
  constraint concentric A59 A60
  constraint coincident L66 A59.end
  constraint concentric A59 A61
  constraint coincident L63 A62.end
  constraint concentric A62 A63
  constraint coincident L66 A62.start
  constraint concentric A62 A64
  constraint coincident L81.end A68.centre
  constraint coincident L82.end A65.centre
  constraint coincident L84.end A74.centre
  constraint coincident L83.end A71.centre
  constraint coincident L68 A65.end
  constraint concentric A65 A66
  constraint coincident L71 A65.start
  constraint concentric A65 A67
  constraint coincident L71 A68.end
  constraint concentric A68 A69
  constraint coincident L70 A68.start
  constraint concentric A68 A70
  constraint coincident L70 A71.end
  constraint concentric A71 A72
  constraint coincident L69 A71.start
  constraint concentric A71 A73
  constraint coincident L69 A74.end
  constraint concentric A74 A75
  constraint coincident L68 A74.start
  constraint concentric A74 A76
  constraint coincident L29 L89.start
  constraint perpendicular L24 L89
  constraint perpendicular L89 L90
  constraint coincident L24 L91.end
  constraint perpendicular L90 L91
  constraint midpoint L90 P6
  constraint coincident L3 P6
  constraint perpendicular L3 L92
  constraint perpendicular L92 L93
  constraint perpendicular L3 L94
  constraint perpendicular L94 L95
  constraint midpoint L96 P7
  constraint coincident L3 P7
  constraint perpendicular L3 L97
  constraint perpendicular L97 L98
  constraint perpendicular L3 L99
  constraint perpendicular L99 L100
  constraint midpoint L101 P8
  constraint coincident L3 P8
  constraint coincident L102.end A86.centre
  constraint coincident L103.end A83.centre
  constraint coincident L105.end A80.centre
  constraint coincident L104.end A77.centre
  constraint coincident L98 A77.end
  constraint concentric A77 A78
  constraint coincident L99 A77.start
  constraint concentric A77 A79
  constraint coincident L98 A80.start
  constraint concentric A80 A81
  constraint coincident L97 A80.end
  constraint concentric A80 A82
  constraint coincident L97 A83.start
  constraint concentric A83 A84
  constraint coincident L100 A83.end
  constraint concentric A83 A85
  constraint coincident L100 A86.start
  constraint concentric A86 A87
  constraint coincident L99 A86.end
  constraint concentric A86 A88
  constraint coincident L113.end A95.centre
  constraint coincident L112.end A98.centre
  constraint coincident L110.end A89.centre
  constraint coincident L111.end A92.centre
  constraint coincident L94 A89.end
  constraint concentric A89 A90
  constraint coincident L95 A89.start
  constraint concentric A89 A91
  constraint coincident L95 A92.end
  constraint concentric A92 A93
  constraint coincident L92 A92.start
  constraint concentric A92 A94
  constraint coincident L92 A95.end
  constraint concentric A95 A96
  constraint coincident L93 A95.start
  constraint concentric A95 A97
  constraint coincident L93 A98.end
  constraint concentric A98 A99
  constraint coincident L94 A98.start
  constraint concentric A98 A100
  constraint horizontal L118
  constraint vertical L119
  constraint horizontal L120
  constraint vertical L121
  constraint coincident A27 L119.end
  constraint coincident A27 L118.end
  constraint horizontal L122
  constraint vertical L123
  constraint horizontal L124
  constraint vertical L125
  constraint coincident A27 L123.end
  constraint coincident A27 L122.end
  constraint coincident L122 L126.start
  constraint coincident L124 L126.end
  constraint perpendicular L124 L126
  constraint coincident L126 L127.start
  constraint coincident A27 L127.end
  constraint coincident L126 L128.start
  constraint coincident A27 L128.end
  constraint coincident L129.end A101.centre
  constraint coincident L120.end A101
  constraint coincident L130.end A102.centre
  constraint coincident L124.end A102
  constraint tangent L120 A103
  constraint tangent L125 A103
  constraint coincident L132.end A104.centre
  constraint coincident L122.start A104
  constraint coincident L131.end A105.centre
  constraint coincident L118.start A105
  constraint tangent L118 A106
  constraint tangent L125 A106
  constraint tangent L128 A107
  constraint tangent A27 A107
  constraint tangent L127 A108
  constraint tangent A27 A108
  constraint tangent L122 A109
  constraint tangent L127 A109
  constraint tangent L124 A110
  constraint tangent L128 A110
  constraint coincident L121 L133.start
  constraint coincident A105 L133.start
  constraint coincident L121 L133.end
  constraint coincident A101 L133.end
  constraint coincident L120 L134.start
  constraint coincident A101 L134.start
  constraint coincident A103 L134.end
  constraint tangent A103 L134
  constraint coincident A103 L135.start
  constraint coincident A102 L135.end
  constraint coincident L125 L135.end
  constraint tangent A103 L135
  constraint coincident L124 L136.start
  constraint coincident A102 L136.start
  constraint coincident A110 L136.end
  constraint tangent A110 L136
  constraint coincident L128 L137.start
  constraint coincident A110 L137.start
  constraint coincident A107 L137.end
  constraint tangent A107 L137
  constraint coincident L118 L138.start
  constraint coincident A105 L138.start
  constraint coincident L118 L138.end
  constraint coincident A106 L138.end
  constraint coincident L125 L139.start
  constraint coincident A106 L139.start
  constraint coincident L125 L139.end
  constraint coincident A104 L139.end
  constraint coincident L122 L140.start
  constraint coincident A104 L140.start
  constraint coincident L122 L140.end
  constraint coincident A109 L140.end
  constraint coincident L127 L141.start
  constraint coincident A109 L141.start
  constraint coincident A108 L141.end
  constraint tangent A108 L141
  constraint coincident A106.centre A115.centre
  constraint coincident A103.centre A116.centre
  constraint coincident A109.centre A117.centre
  constraint coincident A110.centre A118.centre
  constraint coincident A107.centre L142.end
  constraint coincident A27 L143.end
  constraint coincident A107 L143.end
  constraint parallel L142 L143
  constraint coincident A108.centre L144.end
  constraint coincident A108 L145.end
  constraint parallel L144 L145
  constraint coincident L146.end A123.centre
  constraint tangent A121 A123
  constraint tangent L137 A123
  constraint concentric A123 A124
  constraint coincident L147.end A125.centre
  constraint tangent A27 A125
  constraint tangent L28 A125
  constraint concentric A125 A126
  constraint coincident L148.end A127.centre
  constraint tangent L30 A127
  constraint tangent A28 A127
  constraint concentric A127 A128
  constraint coincident L149.end A129.centre
  constraint tangent A28 A129
  constraint tangent L12 A129
  constraint concentric A129 A130
  constraint coincident L150.end A131.centre
  constraint tangent L10 A131
  constraint tangent A25 A131
  constraint concentric A131 A132
  constraint coincident L151.end A133.centre
  constraint tangent A25 A133
  constraint tangent L21 A133
  constraint concentric A133 A134
  constraint coincident L152.end A135.centre
  constraint tangent A122 A135
  constraint tangent L19 A135
  constraint concentric A135 A136
  constraint coincident L153.end A137.centre
  constraint tangent A122 A137
  constraint tangent L141 A137
  constraint concentric A137 A138
  constraint midpoint L155 P9
  constraint midpoint L154 P10
  constraint coincident P10 L156.end
  constraint perpendicular L154 L157
  constraint coincident L157.end A139.centre
  constraint tangent A28 A139
  constraint concentric A139 A140
  constraint coincident P9 L158.end
  constraint perpendicular L155 L159
  constraint coincident L159.end A141.centre
  constraint tangent A25 A141
  constraint concentric A141 A142
  constraint parallel L24 L160
  constraint coincident A28 L161.end
  constraint perpendicular L24 L161